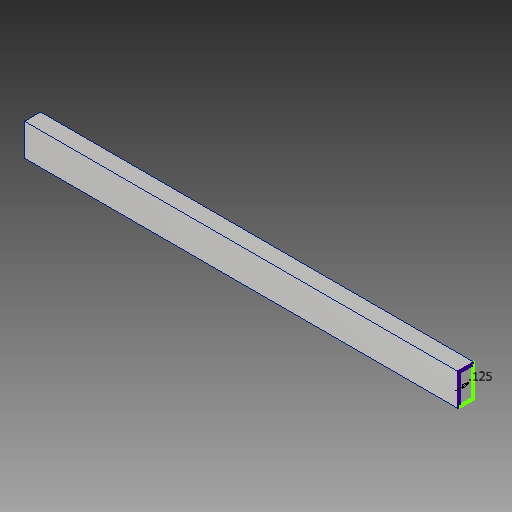
# Autodesk Inventor part: 27inchbarchassis
Saved by Autodesk Inventor 2019 (Build 230136000, 136)
## iProperties
Created: 2019-01-12
Part Number: 27inchbarchassis
Material: Aluminum 6061
Document SubType Name: Modeling
Designer: lebraddock
Density: 2.7 g/cm^3
Appearance: Aluminum - Flat
Mass: 2389.23 g
Surface Area: 1070.97 cm^2
Volume: 884.901 cm^3
Author: lebraddock
Autodesk Inventor part; units mm, degrees
ref_plane "YZ Plane" through (0, 0, 0) normal (1, 0, 0) x (0, 1, 0)
ref_plane "XZ Plane" through (0, 0, 0) normal (0, 1, 0) x (-1, 0, 0)
ref_plane "XY Plane" through (0, 0, 0) normal (0, 0, 1) x (1, 0, 0)
sketch "Sketch1" plane through (0, 0, 0) normal (0, 0, 1) x (1, 0, 0)
  line L0 (-342.9, -25.4) -> (342.9, -25.4)
  line L1 (342.9, -25.4) -> (342.9, 25.4)
  line L2 (342.9, 25.4) -> (-342.9, 25.4)
  line L3 (-342.9, 25.4) -> (-342.9, -25.4)
  line L4 (-342.9, -25.4) -> (342.9, 25.4) construction
  line L5 (342.9, -25.4) -> (-342.9, 25.4) construction
  point P0 (0, 0)
  dimension "d0" = 685.8
  dimension "d1" = 50.8
  constraints: 12 end point, 2 midpoint, 2 parallel, 1 horizontal, 1 perpendicular
  measures "d0" distance of L2.end L1.end
  measures "d1" distance of L1.end L0.end
extrude "Extrusion1" add sketch "Sketch1" along normal blind 25.4
sketch "Sketch2" plane through (342.9, -25.4, 0) normal (1, 0, 0) x (0, 0, -1)
  line L0 (0, 50.8) -> (-25.4, 50.8) projected
  line L1 (-25.4, 50.8) -> (0, 50.8)
  line L2 (0, 50.8) -> (0, 0)
  line L3 (0, 0) -> (-25.4, 0)
  line L4 (-25.4, 0) -> (-25.4, 50.8)
  line L5 (-3.175, 3.175) -> (-3.175, 47.625)
  line L6 (-3.175, 47.625) -> (-22.225, 47.625)
  line L7 (-22.225, 47.625) -> (-22.225, 3.175)
  line L8 (-22.225, 3.175) -> (-3.175, 3.175)
  point P0 (0, 25.4)
  dimension "d4" = 3.175
  constraints: 16 end point, 4 parallel, 2 perpendicular, 1 horizontal, 3 other
  measures "d4" distance between parallel lines of L2 L5
body "Solid1"
